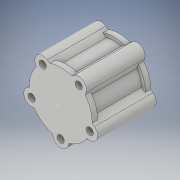
# Autodesk Inventor part: inner
Saved by Autodesk Inventor 2018 (Build 220112000, 112)
## iProperties
Created: 2021-03-12
Part Number: inner
Material: Generic
Document SubType Name: Modeling
Designer: Jyoti Soni
Density: 1 g/cm^3
Appearance: Default
Author: Jyoti Soni
Autodesk Inventor part; units mm, degrees
ref_plane "YZ Plane" through (0, 0, 0) normal (1, 0, 0) x (0, 1, 0)
ref_plane "XZ Plane" through (0, 0, 0) normal (0, 1, 0) x (-1, 0, 0)
ref_plane "XY Plane" through (0, 0, 0) normal (0, 0, 1) x (1, 0, 0)
sketch "Sketch1" plane through (0, 0, 0) normal (0, 0, 1) x (1, 0, 0)
  circle A0 centre (0, 0) radius 77
  dimension "d0" = 154
  constraints: 1 centre point, 1 coincident
  measures "d0" diameter of A0
extrude "Extrusion1" add sketch "Sketch1" along normal blind 162.5
shell "Shell1" thickness 6 removed faces 1 at (-19.0407, -8.1278, 0)
sketch "Sketch2" plane through (0, 0, 162.5) normal (0, 0, 1) x (1, 0, 0)
  circle A0 centre (0, 0) radius 87
  circle A1 centre (0, 0) radius 77
  dimension "d4" = 174
  dimension "d5" = 154
  constraints: 2 centre point, 2 coincident
  measures "d4" diameter of A0
  measures "d5" diameter of A1
extrude "Extrusion2" add sketch "Sketch2" against normal blind 15
sketch "Sketch3" plane through (0, 0, 0) normal (0, 0, -1) x (-1, 0, 0)
  circle A0 centre (0, 0) radius 77 projected
  circle A1 centre (0, 0) radius 87 projected
extrude "Extrusion3" add sketch "Sketch3" against normal blind 15
sketch "Sketch4" plane through (0, 0, 0) normal (0, 0, -1) x (-1, 0, 0)
  arc A0 (70.6417, 62.0029) -> (37.1388, 86.3442) centre (49.9617, 68.7664) ccw
  line L0 (45.2595, 62.2943) -> (49.9617, 68.7664) construction
  line L1 (0, 77) -> (0, 87) construction
  line L2 (70.6417, 62.0029) -> (64.2451, 42.4448)
  arc A1 (68.0794, 54.1683) -> (30.4794, 81.4862) centre (0, 0) ccw construction
  arc A2 (68.0794, 54.1683) -> (30.4794, 81.4862) centre (0, 0) ccw construction
  circle A3 centre (0, 0) radius 77 construction
  circle A4 centre (0, 0) radius 77 construction
  arc A5 (64.2451, 42.4448) -> (-30.3958, 70.7467) centre (0, 0) ccw construction
  arc A6 (64.2451, 42.4448) -> (20.5146, 74.2169) centre (0, 0) ccw
  line L3 (20.5146, 74.2169) -> (37.1388, 86.3442)
  line L4 (76.9238, 3.4237) -> (93.5948, -8.6392)
  arc A7 (80.7978, -48.0243) -> (93.5948, -8.6392) centre (80.8398, -26.2664) ccw
  line L5 (80.7978, -48.0243) -> (60.2203, -47.9846)
  arc A8 (60.2203, -47.9846) -> (57.8913, 50.77) centre (0, 0) ccw construction
  line L6 (27.0269, -72.1009) -> (20.706, -91.6836)
  arc A9 (-20.706, -91.6836) -> (20.706, -91.6836) centre (0, -85) ccw
  line L7 (-20.706, -91.6836) -> (-27.0269, -72.1009)
  arc A10 (-27.0269, -72.1009) -> (66.1746, -39.3691) centre (0, 0) ccw construction
  line L8 (-60.2203, -47.9846) -> (-80.7978, -48.0243)
  arc A11 (-93.5948, -8.6392) -> (-80.7978, -48.0243) centre (-80.8398, -26.2664) ccw
  line L9 (-93.5948, -8.6392) -> (-76.9238, 3.4237)
  arc A12 (-76.9238, 3.4237) -> (-16.9932, -75.1015) centre (0, 0) ccw construction
  line L10 (-64.2451, 42.4448) -> (-70.6417, 62.0029)
  arc A13 (-37.1388, 86.3442) -> (-70.6417, 62.0029) centre (-49.9617, 68.7664) ccw
  line L11 (-37.1388, 86.3442) -> (-20.5146, 74.2169)
  arc A14 (-20.5146, 74.2169) -> (-76.6769, -7.0462) centre (0, 0) ccw construction
  point P0 (72.5548, -48.0084)
  point P1 (-23.2381, -83.8391)
  point P2 (-86.9167, -3.807)
  point P3 (-30.4794, 81.4862)
  dimension "d11" = 85
  dimension "d12" = 36
  dimension "d17" = 360
  constraints: 35 point on circle, 24 end point, 13 centre point, 5 point on line, 3 tangent, 2 coincident, 2 symmetric about line, 1 vertical, 68 other
  measures "d11" distance of point (0, 0) L0.end
  measures "d12" angle of L1 L0
extrude "Extrusion4" add sketch "Sketch4" against normal blind 162.5
pattern_circular "Circular Pattern1" count 5 over 360 about axis through (0, 0, 0) along (0, 0, 1) of "Extrusion4"
sketch "Sketch5" plane through (0, 0, 0) normal (0, 0, -1) x (-1, 0, 0)
  arc A0 (70.6417, 62.0029) -> (37.1388, 86.3442) centre (49.9617, 68.7664) ccw construction
  circle A1 centre (49.9617, 68.7664) radius 10
  point P0 (0, 0)
  dimension "d22" = 20
  constraints: 1 centre point, 1 coincident
  measures "d22" diameter of A1
extrude "Extrusion5" cut sketch "Sketch5" against normal up to next
pattern_circular "Circular Pattern2" count 5 over 360 about axis through (0, 0, 0) along (0, 0, 1) of "Extrusion5"
body "Solid1"
